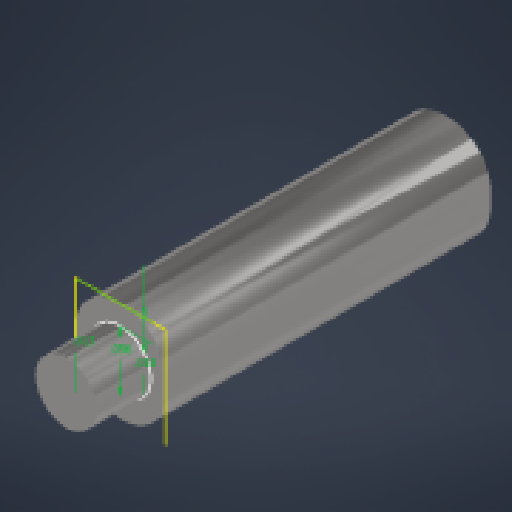
# Autodesk Inventor part: leg
Saved by Autodesk Inventor 2027 (Build 310192000, 192)
## iProperties
Created: 2026-04-24
Part Number: leg
Material: Generic
Document SubType Name: Modeling
Designer: sisis
Density: 1 g/cm^3
Appearance: Default
Author: sisis
Autodesk Inventor part; units mm, degrees
ref_plane "YZ Plane" through (0, 0, 0) normal (1, 0, 0) x (0, 1, 0)
ref_plane "XZ Plane" through (0, 0, 0) normal (0, 1, 0) x (-1, 0, 0)
ref_plane "XY Plane" through (0, 0, 0) normal (0, 0, 1) x (1, 0, 0)
sketch "Sketch1" plane through (0, 0, 0) normal (0, 0, 1) x (1, 0, 0)
  line L0 (0, 2.3308) -> (2.1115, 2.3308)
  line L1 (2.1115, 2.3308) -> (2.1115, 0)
  line L2 (2.1115, 0) -> (0, 0)
  line L3 (0, 0) -> (0, 2.3308)
  constraints: 8 end point, 3 perpendicular, 1 horizontal
extrude "Extrusion1" add sketch "Sketch1" along normal blind 7.62
sketch "Sketch2" plane through (0, 0, 7.62) normal (0, 0, 1) x (1, 0, 0)
  line L0 (2.1115, 2.3308) -> (0, 2.3308) projected
  line L1 (2.1115, 0) -> (2.1115, 2.3308) projected
  line L2 (0, 2.3308) -> (0, 0) projected
  circle A0 centre (1.0558, 1.1654) radius 0.7145
  dimension "d8" = 1.4291
  dimension "d9" = 0.4509
  dimension "d10" = 0.3412
  constraints: 1 centre point
  measures "d8" diameter of A0
  measures "d9" distance edge to line of A0 L0
  measures "d10" distance edge to line of A0 L2
extrude "Extrusion3" add sketch "Sketch2" along normal blind 1.27
fillet "Fillet1" radius 1.016 1 edges at (0, 0, 3.81)
fillet "Fillet2" radius 1.016 1 edges at (2.1115, 0, 3.81)
fillet "Fillet3" radius 1.016 1 edges at (2.1115, 2.3308, 3.81)
fillet "Fillet4" radius 1.016 1 edges at (0, 2.3308, 3.81)
body "Solid1"
